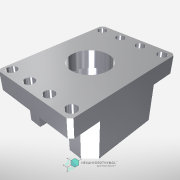
# Autodesk Inventor part: Y-servo-flange
Saved by Autodesk Inventor 2016 (Build 200138000, 138)
## iProperties
Created: 2015-05-21
Part Number: Y-servo-flange
Material: Aluminum 6061-AHC
Document SubType Name: Modeling
Designer: as
Mass: 206.884 g
Surface Area: 203.494 cm^2
Volume: 76.6238 cm^3
Density: 2.7 g/cm^3
Appearance: Aluminum - Dark
Author: as
Autodesk Inventor part; units mm, degrees
ref_plane "YZ Plane" through (0, 0, 0) normal (1, 0, 0) x (0, 1, 0)
ref_plane "XZ Plane" through (0, 0, 0) normal (0, 1, 0) x (-1, 0, 0)
ref_plane "XY Plane" through (0, 0, 0) normal (0, 0, 1) x (1, 0, 0)
sketch "Sketch1" plane through (0, 0, 0) normal (0, 0, 1) x (1, 0, 0)
  line L0 (-27.5, 27.5) -> (27.5, 27.5)
  line L1 (27.5, 27.5) -> (27.5, -27.5)
  line L2 (27.5, -27.5) -> (-27.5, -27.5)
  line L3 (-27.5, -27.5) -> (-27.5, 27.5)
  line L4 (-27.5, 27.5) -> (27.5, -27.5) construction
  line L5 (27.5, 27.5) -> (-27.5, -27.5) construction
  point P0 (0, 0)
  dimension "d0" = 55
  dimension "d1" = 55
  constraints: 12 end point, 2 midpoint, 2 parallel, 1 horizontal, 1 perpendicular
  measures "d0" distance of L1.end L2.end
  measures "d1" distance of L0.end L1.end
extrude "Extrusion1" add sketch "Sketch1" along normal blind 25
sketch "Sketch2" plane through (0, 0, 25) normal (0, 0, 1) x (1, 0, 0)
  line L0 (27.5, 39) -> (-27.5, 39)
  line L1 (-27.5, 39) -> (-27.5, -39)
  line L2 (-27.5, -39) -> (27.5, -39)
  line L3 (27.5, -39) -> (27.5, 39)
  line L4 (27.5, 39) -> (-27.5, -39) construction
  line L5 (-27.5, 39) -> (27.5, -39) construction
  point P0 (0, 0)
  dimension "d4" = 55
  dimension "d5" = 78
  constraints: 12 end point, 2 midpoint, 2 parallel, 1 horizontal, 1 perpendicular
  measures "d4" distance of L2.end L1.end
  measures "d5" distance of L1.end L0.end
extrude "Extrusion2" add sketch "Sketch2" along normal blind 11.5
sketch "Sketch3" plane through (0, 0, 36.5) normal (0, 0, 1) x (1, 0, 0)
  circle A0 centre (0, 0) radius 13
  constraints: 1 centre point, 1 coincident
extrude "Extrusion3" cut sketch "Sketch3" against normal through all
sketch "Sketch4" plane through (0, 0, 36.5) normal (0, 0, 1) x (1, 0, 0)
  line L0 (27.5, -39) -> (27.5, 39) projected
  line L1 (27.5, 39) -> (-27.5, 39) projected
  line L2 (-27.5, 39) -> (-27.5, -39) projected
  line L3 (-27.5, -39) -> (27.5, -39) projected
  point P0 (0, 0)
  point P1 (22.5, 33.5)
  point P2 (22.5, -33.5)
  point P3 (7.5, 33.5)
  point P4 (7.5, -33.5)
  point P5 (-7.5, 33.5)
  point P6 (-7.5, -33.5)
  point P7 (-22.5, 33.5)
  point P8 (-22.5, -33.5)
  dimension "d10" = 5
  dimension "d11" = 5.5
  dimension "d14" = 67
  dimension "d17" = 15
  dimension "d20" = 5
  dimension "d21" = 5.5
  constraints: 1 horizontal, 1 vertical, 7 other
  measures "d10" distance from line of L0 point (22.5, 33.5)
  measures "d11" distance from line of L1 point (22.5, 33.5)
  measures "d14" distance of point (22.5, 33.5) point (22.5, -33.5)
  measures "d17" distance of point (22.5, 33.5) point (7.5, 33.5)
  measures "d20" distance from line of L2 point (-22.5, 33.5)
  measures "d21" distance from line of point (22.5, -33.5) L3
hole "Hole1" at (22.5, 33.5, 36.5) at (22.5, -33.5, 36.5) at (7.5, 33.5, 36.5) at (7.5, -33.5, 36.5) at (-7.5, 33.5, 36.5) at (-7.5, -33.5, 36.5) at (-22.5, 33.5, 36.5) at (-22.5, -33.5, 36.5) direction (0, 0, -1) diameter 6.5 end through all
sketch "Sketch6" plane through (0, 0, 0) normal (0, 0, -1) x (-1, 0, 0)
  circle A0 centre (0, 0) radius 20
  dimension "d40" = 40
  constraints: 1 centre point, 1 coincident
  measures "d40" diameter of A0
extrude "Extrusion5" cut sketch "Sketch6" against normal blind 25
chamfer "Chamfer1" distance 6.5 angle 45 4 edges at (27.5, -27.5, 12.5) (-27.5, -27.5, 12.5) (-27.5, 27.5, 12.5) (27.5, 27.5, 12.5)
chamfer "Chamfer2" distance 2 angle 45 4 edges at (27.5, -39, 30.75) (-27.5, -39, 30.75) (27.5, 39, 30.75) (-27.5, 39, 30.75)
sketch "Sketch5" plane through (-21, -27.5, 0) normal (0, -1, 0) x (1, 0, 0)
  line L0 (42, 0) -> (0, 0) projected
  line L1 (0, 25) -> (42, 25) projected
  line L2 (8.5, 0) -> (33.5, 0)
  line L3 (33.5, 0) -> (33.5, 25)
  line L4 (33.5, 25) -> (8.5, 25)
  line L5 (8.5, 25) -> (8.5, 0)
  point P0 (21, 0)
  dimension "d35" = 25
  dimension "d36" = 12.5
  dimension "d37" = 12.5
  constraints: 8 end point, 2 parallel, 2 point on line, 1 horizontal, 1 perpendicular
  measures "d35" distance of L4.end L3.end
  measures "d36" distance from line of point (21, 0) L5
  measures "d37" distance of point (21, 0) L2.end
extrude "Extrusion4" cut sketch "Sketch5" against normal blind 28
equation "\"d4\" = d0"
body "Solid1"
